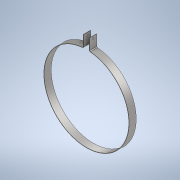
# Autodesk Inventor part: Banda de montaje
Saved by Autodesk Inventor 2021 (Build 250183000, 183)
## iProperties
Created: 2021-07-11
Part Number: Banda de montaje
Material: Generic
Document SubType Name: Modeling
Designer: Nelson
Density: 1 g/cm^3
Appearance: Stainless - Brushed
Author: Nelson
Autodesk Inventor part; units mm, degrees
ref_plane "YZ Plane" through (0, 0, 0) normal (1, 0, 0) x (0, 1, 0)
ref_plane "XZ Plane" through (0, 0, 0) normal (0, 1, 0) x (-1, 0, 0)
ref_plane "XY Plane" through (0, 0, 0) normal (0, 0, 1) x (1, 0, 0)
sketch "Sketch1" plane through (0, 0, 0) normal (0, 0, 1) x (1, 0, 0)
  line L0 (0, 0) -> (0, 19.8871) construction
  arc A0 (-8.2703, 89.6192) -> (8.2703, 89.6192) centre (0, 0) ccw
  arc A1 (-8.353, 90.5154) -> (8.353, 90.5154) centre (0, 0) ccw
  line L1 (-6, 114.7862) -> (-6, 92.1086)
  arc A2 (-8.2703, 89.6192) -> (-6, 92.1086) centre (-8.5, 92.1086) ccw
  arc A3 (-8.353, 90.5154) -> (-6.9, 92.1086) centre (-8.5, 92.1086) ccw
  line L2 (-6.9, 92.1086) -> (-6.9, 114.7862)
  line L3 (-6.9, 114.7862) -> (-6, 114.7862)
  line L4 (6, 114.7862) -> (6, 92.1086)
  arc A4 (6, 92.1086) -> (8.2703, 89.6192) centre (8.5, 92.1086) ccw
  arc A5 (6.9, 92.1086) -> (8.353, 90.5154) centre (8.5, 92.1086) ccw
  line L5 (6.9, 92.1086) -> (6.9, 114.7862)
  line L6 (6.9, 114.7862) -> (6, 114.7862)
  point P0 (-6.455, 90.6705)
  point P1 (6.455, 90.6705)
  dimension "d28" = 180
  dimension "d29" = 181.8
  dimension "d32" = 5
  dimension "d33" = 6
  dimension "d34" = 0.9
  constraints: 14 end point, 14 point on circle, 8 symmetric about line, 6 centre point, 2 coincident, 2 tangent, 2 vertical, 1 horizontal, 3 other
  measures "d28" diameter of A0
  measures "d29" diameter of A1
  measures "d32" diameter of A2
  measures "d33" distance from line of L0.start L1
  measures "d34" radial gap between concentric circles of A2 A3
extrude "Extrusion1" add sketch "Sketch1" against normal blind 15
sketch "Sketch2" plane through (-6.9, 92.1086, 0) normal (-1, 0, 0) x (0, 0, 1)
  line L0 (0, 22.6776) -> (-15, 22.6776) projected
  line L1 (0, 22.6776) -> (0, 0) projected
  point P0 (0, -92.1086)
  point P1 (-7.5, 17.8776)
  dimension "d35" = 4.8
  dimension "d43" = 7.5
  measures "d35" distance from line of L0 point (-7.5, 17.878)
  measures "d43" distance from line of L1 point (-7.5, 17.878)
hole "Hole1" at (-6.9, 109.9862, -7.5) direction (1, 0, 0) diameter 4 depth 25 tip angle 137
body "Solid1"
